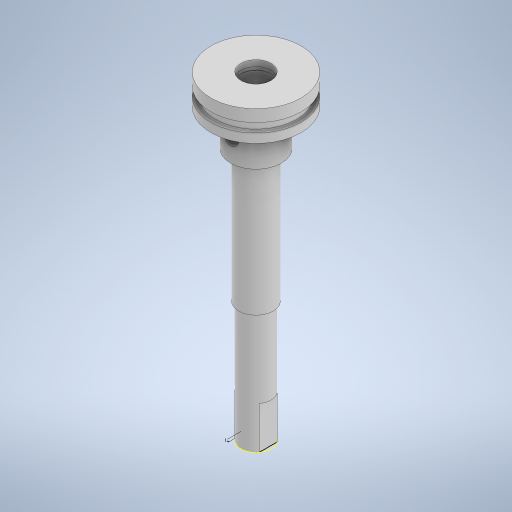
# Autodesk Inventor part: 04-03-2023
Saved by Autodesk Inventor 2023 (Build 270158000, 158)
## iProperties
Created: 2023-04-03
Part Number: 04-03-2023
Material: Generico
Document SubType Name: Modeling
Designer: Admin
Density: 1 g/cm^3
Appearance: Default
Author: Admin
Autodesk Inventor part; units mm, degrees
ref_plane "YZ Plane" through (0, 0, 0) normal (1, 0, 0) x (0, 1, 0)
ref_plane "XZ Plane" through (0, 0, 0) normal (0, 1, 0) x (-1, 0, 0)
ref_plane "XY Plane" through (0, 0, 0) normal (0, 0, 1) x (1, 0, 0)
sketch "Schizzo1" plane through (0, 0, 0) normal (0, 0, 1) x (1, 0, 0)
  line L0 (0, 0) -> (5, 0)
  line L1 (5, 0) -> (5, 40)
  line L2 (5, 40) -> (5.75, 40)
  line L3 (5.75, 40) -> (5.75, 84)
  line L4 (5.75, 84) -> (8.5, 84)
  line L5 (8.5, 84) -> (8.5, 96)
  line L6 (8.5, 96) -> (15, 96)
  line L7 (15, 96) -> (15, 99)
  line L8 (15, 99) -> (13.45, 99)
  line L9 (13.45, 99) -> (13.45, 102)
  line L10 (13.45, 102) -> (15, 102)
  line L11 (15, 102) -> (15, 106)
  line L12 (15, 106) -> (5, 106)
  line L13 (5, 106) -> (5, 104)
  line L14 (5, 104) -> (5.2, 104)
  line L15 (5.2, 104) -> (5.2, 102.9)
  line L16 (5.2, 102.9) -> (5, 102.9)
  line L17 (5, 102.9) -> (5, 96)
  line L18 (5, 96) -> (2.8047, 93.8047)
  line L19 (2.8047, 93.8047) -> (2.8047, 82)
  line L20 (2.8047, 82) -> (0, 80.3148)
  line L21 (0, 80.3148) -> (0, 0)
  dimension "d1" = 10
  dimension "d2" = 11.5
  dimension "d3" = 30
  dimension "d4" = 26.9
  dimension "d5" = 10.4
  dimension "d6" = 10
  dimension "d7" = 5.6094
  dimension "d8" = 17
  dimension "d9" = 40
  dimension "d10" = 84
  dimension "d11" = 96
  dimension "d12" = 10
  dimension "d13" = 4
  dimension "d14" = 3
  dimension "d15" = 2
  dimension "d16" = 1.1
  dimension "d17" = 45
  dimension "d18" = 59
  dimension "d19" = 24
  constraints: 44 end point, 14 perpendicular, 5 point on line, 2 horizontal, 2 parallel
  measures "d1" diameter of L1 L21
  measures "d2" diameter of L3 L21
  measures "d3" diameter of L11 L21
  measures "d4" diameter of L9 L21
  measures "d5" diameter of L15 L21
  measures "d6" diameter of L13 L21
  measures "d7" diameter of L19 L21
  measures "d8" diameter of L5 L21
  measures "d9" distance of L0.end L1.end
  measures "d10" vertical distance of L0.start L3.end
  measures "d11" vertical distance of L0.start L6.end
  measures "d12" distance between parallel lines of L6 L12
  measures "d13" distance of L10.end L11.end
  measures "d14" distance of L8.end L9.end
  measures "d15" distance of L12.end L13.end
  measures "d16" distance of L14.end L15.end
  measures "d17" angle of L19 L18
  measures "d18" angle of L21 L20
  measures "d19" distance from line of L12 L19.end
revolve "Rivoluzione1" add sketch "Schizzo1" angle 360 about axis through (0, 80.3148, 0) along (0, -1, 0)
sketch "Schizzo2" plane through (0, 0, 0) normal (0, 0, 1) x (1, 0, 0)
  circle A0 centre (0, 91.5) radius 2.5
  line L0 (-15, 96) -> (15, 96) projected
  point P0 (0, 0)
  dimension "d21" = 5
  dimension "d22" = 4.5
  constraints: 1 centre point, 1 vertical alignment
  measures "d21" diameter of A0
  measures "d22" distance from line of A0.centre L0
extrude "Estrusione1" cut sketch "Schizzo2" along normal mid plane 30
sketch "Schizzo3" plane through (0, 0, 0) normal (0, -1, 0) x (1, 0, 0)
  line L0 (-4, 3) -> (-4, -3)
  line L1 (4, 3) -> (4, -3)
  circle A0 centre (0, 0) radius 5 projected
  dimension "d25" = 1
  constraints: 4 end point, 4 point on circle, 2 parallel, 1 vertical
  measures "d25" distance edge to line of A0 L0
extrude "Estrusione2" cut sketch "Schizzo3" against normal blind 14 contours L0 A0 | A0 L1
